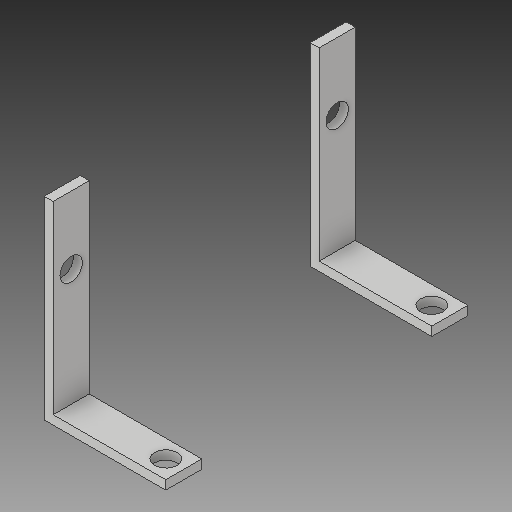
# Autodesk Inventor part: Fixação Caixa de Segurança
Saved by Autodesk Inventor 2019 (Build 230136000, 136)
## iProperties
Created: 2020-05-23
Part Number: Fixação Caixa de Segurança
Material: Genérico
Document SubType Name: Modeling
Designer: lukas
Density: 1 g/cm^3
Appearance: Padrão
Author: lukas
Autodesk Inventor part; units mm, degrees
ref_plane "YZ Plane" through (0, 0, 0) normal (1, 0, 0) x (0, 1, 0)
ref_plane "XZ Plane" through (0, 0, 0) normal (0, 1, 0) x (-1, 0, 0)
ref_plane "XY Plane" through (0, 0, 0) normal (0, 0, 1) x (1, 0, 0)
ref_plane "Plano de trabalho3" through (-51, -1, -36) normal (-1, 0, 0) x (0, 0, 1)
sketch "Esboço7" plane through (-51, -1, -36) normal (-1, 0, 0) x (0, 0, 1)
  circle A0 centre (61, 26) radius 2.5 projected
  line L0 (58.5, 26) -> (58.5, 41)
  line L1 (58.5, 41) -> (57, 41)
  line L2 (57, 41) -> (65, 41)
  line L3 (65, 41) -> (65, -2)
  line L4 (65, -2) -> (57, -2)
  line L5 (57, -2) -> (57, 41)
  line L6 (31.466, 36) -> (31.466, -3.986)
  circle A1 centre (1.932, 26) radius 2.5
  line L7 (5.932, 41) -> (-2.068, 41)
  line L8 (-2.068, 41) -> (-2.068, -2)
  line L9 (-2.068, -2) -> (5.932, -2)
  line L10 (5.932, -2) -> (5.932, 41)
  point P0 (36, 1)
  dimension "d83" = 15
  dimension "d84" = 1.5
  dimension "d85" = 8
  dimension "d86" = 43
  dimension "d114" = 51.068
  constraints: 22 end point, 5 symmetric about line, 3 vertical, 2 horizontal, 2 parallel, 1 centre point, 1 horizontal alignment, 1 perpendicular, 2 other
  measures "d83" distance of L0.start L0.end
  measures "d84" distance of L0.end L1.end
  measures "d85" distance of L3.end L4.end
  measures "d86" distance of L2.end L3.end
  measures "d114" distance of L4.end L10.start
extrude "Extrusão7" add sketch "Esboço7" along normal blind 2
ref_plane "Plano de trabalho6" through (0, -1, 0) normal (0, -1, 0) x (1, 0, 0)
sketch "Esboço8" plane through (0, -1, 0) normal (0, -1, 0) x (1, 0, 0)
  line L0 (-51, 21) -> (-51, 29) projected
  line L1 (-51, 29) -> (-26, 29)
  line L2 (-26, 29) -> (-26, 21)
  line L3 (-26, 21) -> (-51, 21)
  line L4 (-51, 21) -> (-51, 29)
  line L5 (-51, -38.068) -> (-26, -38.068)
  line L6 (-26, -38.068) -> (-26, -30.068)
  line L7 (-26, -30.068) -> (-51, -30.068)
  line L8 (-51, -30.068) -> (-51, -38.068)
  circle A0 centre (-30, 25) radius 2.5
  circle A1 centre (-30, -34.068) radius 2.5
  line L9 (-26, -34.068) -> (-30, -34.068)
  line L10 (-51, -30.068) -> (-51, -38.068) projected
  line L11 (-26, -30.068) -> (-51, -30.068)
  line L12 (-51, -30.068) -> (-51, -38.068)
  line L13 (-26, -33.136) -> (-26, -30.068)
  line L14 (-26, -30.068) -> (-51, -30.068)
  line L15 (-51, -30.068) -> (-51, -38.068)
  line L16 (-51, -38.068) -> (-26, -38.068)
  line L17 (-26, -38.068) -> (-26, -30.068)
  line L18 (-26, 25) -> (-30, 25)
  line L19 (-51, 29) -> (-26, 29)
  line L20 (-26, 29) -> (-26, 21)
  line L21 (-26, 21) -> (-51, 21)
  line L22 (-51, 21) -> (-51, 29)
  point P0 (0, 0)
  dimension "d89" = 25
  dimension "d90" = 25
  dimension "d115" = 51.068
  dimension "d116" = 4
  dimension "d117" = 4
  constraints: 42 end point, 9 parallel, 7 horizontal, 5 perpendicular, 2 centre point, 2 midpoint
  measures "d89" distance of L2.end L3.end
  measures "d90" distance of L7.end L6.end
  measures "d115" distance of L6.end L2.end
  measures "d116" distance of L9.start L9.end
  measures "d117" distance of L18.start L18.end
extrude "Extrusão8" add sketch "Esboço8" along normal blind 2
